Autodesk Fusion 360 part; units mm, degrees
(part 6 of 7)
  line L308 (64.4437, -54.0323) -> (64.499, -54.1149)
  line L309 (64.499, -54.1149) -> (64.5587, -54.1969)
  line L310 (64.5587, -54.1969) -> (64.6439, -54.1986)
  line L311 (64.6439, -54.1986) -> (64.7292, -54.1986)
  line L312 (64.7292, -54.1986) -> (64.8145, -54.1969)
  line L313 (64.8145, -54.1969) -> (64.8741, -54.1149)
  line L314 (64.8741, -54.1149) -> (64.9295, -54.0323)
  line L315 (64.9295, -54.0323) -> (64.9805, -53.949)
  line L316 (64.9805, -53.949) -> (65.027, -53.8654)
  line L317 (65.027, -53.8654) -> (65.069, -53.7814)
  line L318 (65.069, -53.7814) -> (65.1064, -53.6974)
  line L319 (65.1064, -53.6974) -> (65.1389, -53.6134)
  line L320 (65.1389, -53.6134) -> (65.1663, -53.5295)
  line L321 (65.1663, -53.5295) -> (65.1884, -53.4461)
  line L322 (65.1884, -53.4461) -> (65.2045, -53.3632)
  line L323 (65.2045, -53.3632) -> (65.2136, -53.2811)
  line L324 (65.2136, -53.2811) -> (65.2128, -53.2005)
  line L325 (65.2128, -53.2005) -> (65.1672, -52.9112)
  line L326 (65.1672, -52.9112) -> (65.3277, -52.8816)
  line L327 (65.3277, -52.8816) -> (65.4863, -52.8435)
  line L328 (65.4863, -52.8435) -> (65.6428, -52.7972)
  line L329 (65.6428, -52.7972) -> (65.7965, -52.7426)
  line L330 (65.7965, -52.7426) -> (65.9017, -53.0159)
  line L331 (65.9017, -53.0159) -> (65.9413, -53.0862)
  line L332 (65.9413, -53.0862) -> (65.9903, -53.1526)
  line L333 (65.9903, -53.1526) -> (66.0456, -53.2164)
  line L334 (66.0456, -53.2164) -> (66.1065, -53.2776)
  line L335 (66.1065, -53.2776) -> (66.1721, -53.3365)
  line L336 (66.1721, -53.3365) -> (66.2423, -53.393)
  line L337 (66.2423, -53.393) -> (66.3167, -53.4471)
  line L338 (66.3167, -53.4471) -> (66.395, -53.4988)
  line L339 (66.395, -53.4988) -> (66.4772, -53.548)
  line L340 (66.4772, -53.548) -> (66.563, -53.5946)
  line L341 (66.563, -53.5946) -> (66.6522, -53.6385)
  line L342 (66.6522, -53.6385) -> (66.7449, -53.6797)
  line L343 (66.7449, -53.6797) -> (66.8195, -53.6385)
  line L344 (66.8195, -53.6385) -> (66.8934, -53.5959)
  line L345 (66.8934, -53.5959) -> (66.9664, -53.5518)
  line L346 (66.9664, -53.5518) -> (66.9771, -53.451)
  line L347 (66.9771, -53.451) -> (66.9836, -53.3517)
  line L348 (66.9836, -53.3517) -> (66.9862, -53.2541)
  line L349 (66.9862, -53.2541) -> (66.9847, -53.1584)
  line L350 (66.9847, -53.1584) -> (66.9791, -53.0647)
  line L351 (66.9791, -53.0647) -> (66.9694, -52.9732)
  line L352 (66.9694, -52.9732) -> (66.9556, -52.8842)
  line L353 (66.9556, -52.8842) -> (66.9374, -52.7979)
  line L354 (66.9374, -52.7979) -> (66.9148, -52.7146)
  line L355 (66.9148, -52.7146) -> (66.8873, -52.6347)
  line L356 (66.8873, -52.6347) -> (66.8542, -52.5591)
  line L357 (66.8542, -52.5591) -> (66.8131, -52.4897)
  line L358 (66.8131, -52.4897) -> (66.629, -52.262)
  line L359 (66.629, -52.262) -> (66.7532, -52.1561)
  line L360 (66.7532, -52.1561) -> (66.8715, -52.0438)
  line L361 (66.8715, -52.0438) -> (66.9838, -51.9254)
  line L362 (66.9838, -51.9254) -> (67.0897, -51.8013)
  line L363 (67.0897, -51.8013) -> (67.3175, -51.9854)
  line L364 (67.3175, -51.9854) -> (67.3869, -52.0264)
  line L365 (67.3869, -52.0264) -> (67.4625, -52.0595)
  line L366 (67.4625, -52.0595) -> (67.5423, -52.087)
  line L367 (67.5423, -52.087) -> (67.6256, -52.1097)
  line L368 (67.6256, -52.1097) -> (67.712, -52.1278)
  line L369 (67.712, -52.1278) -> (67.801, -52.1417)
  line L370 (67.801, -52.1417) -> (67.8924, -52.1513)
  line L371 (67.8924, -52.1513) -> (67.9861, -52.1569)
  line L372 (67.9861, -52.1569) -> (68.0819, -52.1584)
  line L373 (68.0819, -52.1584) -> (68.1794, -52.1559)
  line L374 (68.1794, -52.1559) -> (68.2787, -52.1493)
  line L375 (68.2787, -52.1493) -> (68.3795, -52.1387)
  line L376 (68.3795, -52.1387) -> (68.4236, -52.0657)
  line L377 (68.4236, -52.0657) -> (68.4663, -51.9918)
  line L378 (68.4663, -51.9918) -> (68.5075, -51.9171)
  line L379 (68.5075, -51.9171) -> (68.4663, -51.8245)
  line L380 (68.4663, -51.8245) -> (68.4223, -51.7352)
  line L381 (68.4223, -51.7352) -> (68.3757, -51.6494)
  line L382 (68.3757, -51.6494) -> (68.3266, -51.5673)
  line L383 (68.3266, -51.5673) -> (68.2749, -51.4889)
  line L384 (68.2749, -51.4889) -> (68.2208, -51.4146)
  line L385 (68.2208, -51.4146) -> (68.1643, -51.3444)
  line L386 (68.1643, -51.3444) -> (68.1054, -51.2787)
  line L387 (68.1054, -51.2787) -> (68.0441, -51.2179)
  line L388 (68.0441, -51.2179) -> (67.9804, -51.1625)
  line L389 (67.9804, -51.1625) -> (67.9139, -51.1135)
  line L390 (67.9139, -51.1135) -> (67.8437, -51.074)
  line L391 (67.8437, -51.074) -> (67.5704, -50.9688)
  line L392 (67.5704, -50.9688) -> (67.6249, -50.815)
  line L393 (67.6249, -50.815) -> (67.6713, -50.6586)
  line L394 (67.6713, -50.6586) -> (67.7094, -50.4999)
  line L395 (67.7094, -50.4999) -> (67.739, -50.3395)
  circle A0 centre (64.6866, -49.8588) radius 1.5
extrude "Extrude2''" add sketch "Sketch2 (3)" along normal blind 2 separate body makes body 9 in component "CT idler 3"
combine "Combine1''" operation add target body 8 tool bodies 9 makes body 10 at (63.4191, -47.6635, 43.4) in component "CT idler 3"
ref_plane "WorkPlane1" through (0, 0, 43.4) normal (0, 0, 1) x (1, 0, 0) in component "CT dial wheel (tool body)"
sketch "Sketch1 (5)" plane through (0, 0, 43.4) normal (0, 0, 1) x (1, 0, 0) in component "CT dial wheel (tool body)"
  line L0 (77.4997, -64.3893) -> (77.838, -64.4048)
  line L1 (77.838, -64.4048) -> (77.9192, -64.4017)
  line L2 (77.9192, -64.4017) -> (78.0006, -64.3928)
  line L3 (78.0006, -64.3928) -> (78.0822, -64.3801)
  line L4 (78.0822, -64.3801) -> (78.1639, -64.3643)
  line L5 (78.1639, -64.3643) -> (78.2456, -64.3456)
  line L6 (78.2456, -64.3456) -> (78.3274, -64.3244)
  line L7 (78.3274, -64.3244) -> (78.4092, -64.3009)
  line L8 (78.4092, -64.3009) -> (78.491, -64.2751)
  line L9 (78.491, -64.2751) -> (78.5728, -64.2472)
  line L10 (78.5728, -64.2472) -> (78.6546, -64.2173)
  line L11 (78.6546, -64.2173) -> (78.7363, -64.1854)
  line L12 (78.7363, -64.1854) -> (78.818, -64.1516)
  line L13 (78.818, -64.1516) -> (78.8198, -64.0105)
  line L14 (78.8198, -64.0105) -> (78.8198, -63.8695)
  line L15 (78.8198, -63.8695) -> (78.818, -63.7284)
  line L16 (78.818, -63.7284) -> (78.7363, -63.6946)
  line L17 (78.7363, -63.6946) -> (78.6546, -63.6627)
  line L18 (78.6546, -63.6627) -> (78.5728, -63.6328)
  line L19 (78.5728, -63.6328) -> (78.491, -63.6049)
  line L20 (78.491, -63.6049) -> (78.4092, -63.5791)
  line L21 (78.4092, -63.5791) -> (78.3274, -63.5556)
  line L22 (78.3274, -63.5556) -> (78.2456, -63.5344)
  line L23 (78.2456, -63.5344) -> (78.1639, -63.5157)
  line L24 (78.1639, -63.5157) -> (78.0822, -63.4999)
  line L25 (78.0822, -63.4999) -> (78.0006, -63.4872)
  line L26 (78.0006, -63.4872) -> (77.9192, -63.4783)
  line L27 (77.9192, -63.4783) -> (77.838, -63.4752)
  line L28 (77.838, -63.4752) -> (77.4997, -63.4907)
  line L29 (77.4997, -63.4907) -> (77.4883, -63.2877)
  line L30 (77.4883, -63.2877) -> (77.4727, -63.085)
  line L31 (77.4727, -63.085) -> (77.4529, -62.8827)
  line L32 (77.4529, -62.8827) -> (77.4289, -62.6808)
  line L33 (77.4289, -62.6808) -> (77.7647, -62.6373)
  line L34 (77.7647, -62.6373) -> (77.8441, -62.6202)
  line L35 (77.8441, -62.6202) -> (77.9228, -62.5973)
  line L36 (77.9228, -62.5973) -> (78.0009, -62.5706)
  line L37 (78.0009, -62.5706) -> (78.0786, -62.5408)
  line L38 (78.0786, -62.5408) -> (78.1558, -62.5082)
  line L39 (78.1558, -62.5082) -> (78.2327, -62.4731)
  line L40 (78.2327, -62.4731) -> (78.3092, -62.4357)
  line L41 (78.3092, -62.4357) -> (78.3853, -62.3962)
  line L42 (78.3853, -62.3962) -> (78.461, -62.3545)
  line L43 (78.461, -62.3545) -> (78.5363, -62.3108)
  line L44 (78.5363, -62.3108) -> (78.6113, -62.2652)
  line L45 (78.6113, -62.2652) -> (78.6858, -62.2178)
  line L46 (78.6858, -62.2178) -> (78.6631, -62.0785)
  line L47 (78.6631, -62.0785) -> (78.6386, -61.9396)
  line L48 (78.6386, -61.9396) -> (78.6123, -61.801)
  line L49 (78.6123, -61.801) -> (78.526, -61.7819)
  line L50 (78.526, -61.7819) -> (78.44, -61.7647)
  line L51 (78.44, -61.7647) -> (78.3543, -61.7494)
  line L52 (78.3543, -61.7494) -> (78.2689, -61.7362)
  line L53 (78.2689, -61.7362) -> (78.1838, -61.725)
  line L54 (78.1838, -61.725) -> (78.0992, -61.716)
  line L55 (78.0992, -61.716) -> (78.015, -61.7093)
  line L56 (78.015, -61.7093) -> (77.9312, -61.7052)
  line L57 (77.9312, -61.7052) -> (77.848, -61.7037)
  line L58 (77.848, -61.7037) -> (77.7655, -61.7054)
  line L59 (77.7655, -61.7054) -> (77.6838, -61.7108)
  line L60 (77.6838, -61.7108) -> (77.6033, -61.7218)
  line L61 (77.6033, -61.7218) -> (77.2728, -61.7958)
  line L62 (77.2728, -61.7958) -> (77.2263, -61.5979)
  line L63 (77.2263, -61.5979) -> (77.1757, -61.401)
  line L64 (77.1757, -61.401) -> (77.1211, -61.2052)
  line L65 (77.1211, -61.2052) -> (77.0624, -61.0105)
  line L66 (77.0624, -61.0105) -> (77.3856, -60.9094)
  line L67 (77.3856, -60.9094) -> (77.4608, -60.8787)
  line L68 (77.4608, -60.8787) -> (77.5343, -60.8425)
  line L69 (77.5343, -60.8425) -> (77.6066, -60.8027)
  line L70 (77.6066, -60.8027) -> (77.6779, -60.7598)
  line L71 (77.6779, -60.7598) -> (77.7483, -60.7143)
  line L72 (77.7483, -60.7143) -> (77.818, -60.6664)
  line L73 (77.818, -60.6664) -> (77.8868, -60.6163)
  line L74 (77.8868, -60.6163) -> (77.9549, -60.5641)
  line L75 (77.9549, -60.5641) -> (78.0222, -60.5099)
  line L76 (78.0222, -60.5099) -> (78.0888, -60.4539)
  line L77 (78.0888, -60.4539) -> (78.1547, -60.396)
  line L78 (78.1547, -60.396) -> (78.2199, -60.3363)
  line L79 (78.2199, -60.3363) -> (78.1733, -60.2031)
  line L80 (78.1733, -60.2031) -> (78.125, -60.0705)
  line L81 (78.125, -60.0705) -> (78.0751, -59.9386)
  line L82 (78.0751, -59.9386) -> (77.9868, -59.9347)
  line L83 (77.9868, -59.9347) -> (77.8991, -59.9327)
  line L84 (77.8991, -59.9327) -> (77.8121, -59.9326)
  line L85 (77.8121, -59.9326) -> (77.7256, -59.9344)
  line L86 (77.7256, -59.9344) -> (77.6399, -59.9381)
  line L87 (77.6399, -59.9381) -> (77.555, -59.944)
  line L88 (77.555, -59.944) -> (77.4709, -59.9521)
  line L89 (77.4709, -59.9521) -> (77.3877, -59.9625)
  line L90 (77.3877, -59.9625) -> (77.3055, -59.9755)
  line L91 (77.3055, -59.9755) -> (77.2245, -59.9915)
  line L92 (77.2245, -59.9915) -> (77.145, -60.011)
  line L93 (77.145, -60.011) -> (77.0676, -60.0358)
  line L94 (77.0676, -60.0358) -> (76.755, -60.1661)
  line L95 (76.755, -60.1661) -> (76.6749, -59.9792)
  line L96 (76.6749, -59.9792) -> (76.5909, -59.7941)
  line L97 (76.5909, -59.7941) -> (76.5031, -59.6108)
  line L98 (76.5031, -59.6108) -> (76.4115, -59.4293)
  line L99 (76.4115, -59.4293) -> (76.7122, -59.2736)
  line L100 (76.7122, -59.2736) -> (76.7809, -59.2303)
  line L101 (76.7809, -59.2303) -> (76.847, -59.1819)
  line L102 (76.847, -59.1819) -> (76.9113, -59.1301)
  line L103 (76.9113, -59.1301) -> (76.9741, -59.0755)
  line L104 (76.9741, -59.0755) -> (77.0356, -59.0185)
  line L105 (77.0356, -59.0185) -> (77.0958, -58.9592)
  line L106 (77.0958, -58.9592) -> (77.1549, -58.8979)
  line L107 (77.1549, -58.8979) -> (77.2128, -58.8347)
  line L108 (77.2128, -58.8347) -> (77.2697, -58.7696)
  line L109 (77.2697, -58.7696) -> (77.3256, -58.7028)
  line L110 (77.3256, -58.7028) -> (77.3804, -58.6344)
  line L111 (77.3804, -58.6344) -> (77.4343, -58.5643)
  line L112 (77.4343, -58.5643) -> (77.3653, -58.4412)
  line L113 (77.3653, -58.4412) -> (77.2947, -58.319)
  line L114 (77.2947, -58.319) -> (77.2226, -58.1977)
  line L115 (77.2226, -58.1977) -> (77.135, -58.2093)
  line L116 (77.135, -58.2093) -> (77.0483, -58.2226)
  line L117 (77.0483, -58.2226) -> (76.9625, -58.2375)
  line L118 (76.9625, -58.2375) -> (76.8778, -58.2543)
  line L119 (76.8778, -58.2543) -> (76.794, -58.2729)
  line L120 (76.794, -58.2729) -> (76.7114, -58.2934)
  line L121 (76.7114, -58.2934) -> (76.63, -58.3159)
  line L122 (76.63, -58.3159) -> (76.5498, -58.3407)
  line L123 (76.5498, -58.3407) -> (76.4712, -58.3677)
  line L124 (76.4712, -58.3677) -> (76.3942, -58.3975)
  line L125 (76.3942, -58.3975) -> (76.3192, -58.4305)
  line L126 (76.3192, -58.4305) -> (76.2474, -58.4684)
  line L127 (76.2474, -58.4684) -> (75.9621, -58.651)
  line L128 (75.9621, -58.651) -> (75.8508, -58.4809)
  line L129 (75.8508, -58.4809) -> (75.7359, -58.3132)
  line L130 (75.7359, -58.3132) -> (75.6176, -58.1479)
  line L131 (75.6176, -58.1479) -> (75.4958, -57.9851)
  line L132 (75.4958, -57.9851) -> (75.765, -57.7795)
  line L133 (75.765, -57.7795) -> (75.8251, -57.7249)
  line L134 (75.8251, -57.7249) -> (75.8818, -57.6658)
  line L135 (75.8818, -57.6658) -> (75.9361, -57.6036)
  line L136 (75.9361, -57.6036) -> (75.9885, -57.539)
  line L137 (75.9885, -57.539) -> (76.0391, -57.4721)
  line L138 (76.0391, -57.4721) -> (76.0881, -57.4033)
  line L139 (76.0881, -57.4033) -> (76.1357, -57.3327)
  line L140 (76.1357, -57.3327) -> (76.1818, -57.2604)
  line L141 (76.1818, -57.2604) -> (76.2265, -57.1864)
  line L142 (76.2265, -57.1864) -> (76.2699, -57.1109)
  line L143 (76.2699, -57.1109) -> (76.3121, -57.034)
  line L144 (76.3121, -57.034) -> (76.3529, -56.9556)
  line L145 (76.3529, -56.9556) -> (76.2636, -56.8464)
  line L146 (76.2636, -56.8464) -> (76.1729, -56.7383)
  line L147 (76.1729, -56.7383) -> (76.0808, -56.6314)
  line L148 (76.0808, -56.6314) -> (75.9966, -56.658)
  line L149 (75.9966, -56.658) -> (75.9135, -56.6861)
  line L150 (75.9135, -56.6861) -> (75.8316, -56.7158)
  line L151 (75.8316, -56.7158) -> (75.751, -56.747)
  line L152 (75.751, -56.747) -> (75.6718, -56.7798)
  line L153 (75.6718, -56.7798) -> (75.594, -56.8144)
  line L154 (75.594, -56.8144) -> (75.5177, -56.8507)
  line L155 (75.5177, -56.8507) -> (75.4431, -56.889)
  line L156 (75.4431, -56.889) -> (75.3703, -56.9293)
  line L157 (75.3703, -56.9293) -> (75.2997, -56.972)
  line L158 (75.2997, -56.972) -> (75.2316, -57.0175)
  line L159 (75.2316, -57.0175) -> (75.1674, -57.0673)
  line L160 (75.1674, -57.0673) -> (74.9182, -57.2967)
  line L161 (74.9182, -57.2967) -> (74.779, -57.1485)
  line L162 (74.779, -57.1485) -> (74.6367, -57.0033)
  line L163 (74.6367, -57.0033) -> (74.4915, -56.861)
  line L164 (74.4915, -56.861) -> (74.3433, -56.7218)
  line L165 (74.3433, -56.7218) -> (74.5727, -56.4726)
  line L166 (74.5727, -56.4726) -> (74.6225, -56.4084)
  line L167 (74.6225, -56.4084) -> (74.668, -56.3403)
  line L168 (74.668, -56.3403) -> (74.7107, -56.2697)
  line L169 (74.7107, -56.2697) -> (74.751, -56.1969)
  line L170 (74.751, -56.1969) -> (74.7893, -56.1223)
  line L171 (74.7893, -56.1223) -> (74.8256, -56.046)
  line L172 (74.8256, -56.046) -> (74.8602, -55.9682)
  line L173 (74.8602, -55.9682) -> (74.893, -55.889)
  line L174 (74.893, -55.889) -> (74.9242, -55.8084)
  line L175 (74.9242, -55.8084) -> (74.9539, -55.7265)
  line L176 (74.9539, -55.7265) -> (74.982, -55.6434)
  line L177 (74.982, -55.6434) -> (75.0086, -55.5592)
  line L178 (75.0086, -55.5592) -> (74.9017, -55.4671)
  line L179 (74.9017, -55.4671) -> (74.7936, -55.3764)
  line L180 (74.7936, -55.3764) -> (74.6844, -55.2871)
  line L181 (74.6844, -55.2871) -> (74.606, -55.3279)
  line L182 (74.606, -55.3279) -> (74.5291, -55.3701)
  line L183 (74.5291, -55.3701) -> (74.4536, -55.4135)
  line L184 (74.4536, -55.4135) -> (74.3796, -55.4582)
  line L185 (74.3796, -55.4582) -> (74.3073, -55.5043)
  line L186 (74.3073, -55.5043) -> (74.2367, -55.5519)
  line L187 (74.2367, -55.5519) -> (74.1679, -55.6009)
  line L188 (74.1679, -55.6009) -> (74.101, -55.6515)
  line L189 (74.101, -55.6515) -> (74.0364, -55.7039)
  line L190 (74.0364, -55.7039) -> (73.9742, -55.7582)
  line L191 (73.9742, -55.7582) -> (73.9151, -55.8149)
  line L192 (73.9151, -55.8149) -> (73.8605, -55.875)
  line L193 (73.8605, -55.875) -> (73.6549, -56.1442)
  line L194 (73.6549, -56.1442) -> (73.4921, -56.0224)
  line L195 (73.4921, -56.0224) -> (73.3268, -55.9041)
  line L196 (73.3268, -55.9041) -> (73.1591, -55.7892)
  line L197 (73.1591, -55.7892) -> (72.989, -55.6779)
  line L198 (72.989, -55.6779) -> (73.1716, -55.3926)
  line L199 (73.1716, -55.3926) -> (73.2095, -55.3208)
  line L200 (73.2095, -55.3208) -> (73.2425, -55.2458)
  line L201 (73.2425, -55.2458) -> (73.2723, -55.1688)
  line L202 (73.2723, -55.1688) -> (73.2993, -55.0902)
  line L203 (73.2993, -55.0902) -> (73.3241, -55.01)
  line L204 (73.3241, -55.01) -> (73.3466, -54.9286)
  line L205 (73.3466, -54.9286) -> (73.3671, -54.846)
  line L206 (73.3671, -54.846) -> (73.3857, -54.7622)
  line L207 (73.3857, -54.7622) -> (73.4025, -54.6775)
  line L208 (73.4025, -54.6775) -> (73.4174, -54.5917)
  line L209 (73.4174, -54.5917) -> (73.4307, -54.505)
  line L210 (73.4307, -54.505) -> (73.4423, -54.4174)
  line L211 (73.4423, -54.4174) -> (73.321, -54.3453)
  line L212 (73.321, -54.3453) -> (73.1988, -54.2747)
  line L213 (73.1988, -54.2747) -> (73.0757, -54.2057)
  line L214 (73.0757, -54.2057) -> (73.0056, -54.2596)
  line L215 (73.0056, -54.2596) -> (72.9372, -54.3144)
  line L216 (72.9372, -54.3144) -> (72.8704, -54.3703)
  line L217 (72.8704, -54.3703) -> (72.8053, -54.4272)
  line L218 (72.8053, -54.4272) -> (72.7421, -54.4851)
  line L219 (72.7421, -54.4851) -> (72.6808, -54.5442)
  line L220 (72.6808, -54.5442) -> (72.6215, -54.6044)
  line L221 (72.6215, -54.6044) -> (72.5645, -54.6659)
  line L222 (72.5645, -54.6659) -> (72.5099, -54.7287)
  line L223 (72.5099, -54.7287) -> (72.4581, -54.793)
  line L224 (72.4581, -54.793) -> (72.4097, -54.8591)
  line L225 (72.4097, -54.8591) -> (72.3664, -54.9278)
  line L226 (72.3664, -54.9278) -> (72.2107, -55.2285)
  line L227 (72.2107, -55.2285) -> (72.0292, -55.1369)
  line L228 (72.0292, -55.1369) -> (71.8459, -55.0491)
  line L229 (71.8459, -55.0491) -> (71.6608, -54.9651)
  line L230 (71.6608, -54.9651) -> (71.4739, -54.885)
  line L231 (71.4739, -54.885) -> (71.6042, -54.5724)
  line L232 (71.6042, -54.5724) -> (71.629, -54.495)
  line L233 (71.629, -54.495) -> (71.6485, -54.4155)
  line L234 (71.6485, -54.4155) -> (71.6645, -54.3345)
  line L235 (71.6645, -54.3345) -> (71.6775, -54.2523)
  line L236 (71.6775, -54.2523) -> (71.6879, -54.1691)
  line L237 (71.6879, -54.1691) -> (71.696, -54.085)
  line L238 (71.696, -54.085) -> (71.7019, -54.0001)
  line L239 (71.7019, -54.0001) -> (71.7056, -53.9144)
  line L240 (71.7056, -53.9144) -> (71.7074, -53.8279)
  line L241 (71.7074, -53.8279) -> (71.7073, -53.7409)
  line L242 (71.7073, -53.7409) -> (71.7053, -53.6532)
  line L243 (71.7053, -53.6532) -> (71.7014, -53.5649)
  line L244 (71.7014, -53.5649) -> (71.5695, -53.515)
  line L245 (71.5695, -53.515) -> (71.4369, -53.4667)
  line L246 (71.4369, -53.4667) -> (71.3037, -53.4201)
  line L247 (71.3037, -53.4201) -> (71.244, -53.4853)
  line L248 (71.244, -53.4853) -> (71.1861, -53.5512)
  line L249 (71.1861, -53.5512) -> (71.1301, -53.6178)
  line L250 (71.1301, -53.6178) -> (71.0759, -53.6851)
  line L251 (71.0759, -53.6851) -> (71.0237, -53.7532)
  line L252 (71.0237, -53.7532) -> (70.9736, -53.822)
  line L253 (70.9736, -53.822) -> (70.9257, -53.8917)
  line L254 (70.9257, -53.8917) -> (70.8802, -53.9621)
  line L255 (70.8802, -53.9621) -> (70.8373, -54.0334)
  line L256 (70.8373, -54.0334) -> (70.7975, -54.1057)
  line L257 (70.7975, -54.1057) -> (70.7613, -54.1792)
  line L258 (70.7613, -54.1792) -> (70.7306, -54.2544)
  line L259 (70.7306, -54.2544) -> (70.6295, -54.5776)
  line L260 (70.6295, -54.5776) -> (70.4348, -54.5189)
  line L261 (70.4348, -54.5189) -> (70.239, -54.4643)
  line L262 (70.239, -54.4643) -> (70.0421, -54.4137)
  line L263 (70.0421, -54.4137) -> (69.8442, -54.3672)
  line L264 (69.8442, -54.3672) -> (69.9182, -54.0367)
  line L265 (69.9182, -54.0367) -> (69.9292, -53.9562)
  line L266 (69.9292, -53.9562) -> (69.9346, -53.8745)
  line L267 (69.9346, -53.8745) -> (69.9363, -53.792)
  line L268 (69.9363, -53.792) -> (69.9348, -53.7088)
  line L269 (69.9348, -53.7088) -> (69.9307, -53.625)
  line L270 (69.9307, -53.625) -> (69.924, -53.5408)
  line L271 (69.924, -53.5408) -> (69.915, -53.4562)
  line L272 (69.915, -53.4562) -> (69.9038, -53.3711)
  line L273 (69.9038, -53.3711) -> (69.8906, -53.2857)
  line L274 (69.8906, -53.2857) -> (69.8753, -53.2)
  line L275 (69.8753, -53.2) -> (69.8581, -53.114)
  line L276 (69.8581, -53.114) -> (69.839, -53.0277)
  line L277 (69.839, -53.0277) -> (69.7004, -53.0014)
  line L278 (69.7004, -53.0014) -> (69.5615, -52.9769)
  line L279 (69.5615, -52.9769) -> (69.4222, -52.9542)
  line L280 (69.4222, -52.9542) -> (69.3748, -53.0287)
  line L281 (69.3748, -53.0287) -> (69.3292, -53.1037)
  line L282 (69.3292, -53.1037) -> (69.2855, -53.179)
  line L283 (69.2855, -53.179) -> (69.2438, -53.2547)
  line L284 (69.2438, -53.2547) -> (69.2043, -53.3308)
  line L285 (69.2043, -53.3308) -> (69.1669, -53.4073)
  line L286 (69.1669, -53.4073) -> (69.1318, -53.4842)
  line L287 (69.1318, -53.4842) -> (69.0992, -53.5614)
  line L288 (69.0992, -53.5614) -> (69.0694, -53.6391)
  line L289 (69.0694, -53.6391) -> (69.0427, -53.7172)
  line L290 (69.0427, -53.7172) -> (69.0198, -53.7959)
  line L291 (69.0198, -53.7959) -> (69.0027, -53.8753)
  line L292 (69.0027, -53.8753) -> (68.9592, -54.2111)
  line L293 (68.9592, -54.2111) -> (68.7573, -54.1871)
  line L294 (68.7573, -54.1871) -> (68.555, -54.1673)
  line L295 (68.555, -54.1673) -> (68.3523, -54.1517)
  line L296 (68.3523, -54.1517) -> (68.1493, -54.1403)
  line L297 (68.1493, -54.1403) -> (68.1648, -53.802)
  line L298 (68.1648, -53.802) -> (68.1617, -53.7208)
  line L299 (68.1617, -53.7208) -> (68.1528, -53.6394)
  line L300 (68.1528, -53.6394) -> (68.1401, -53.5578)
  line L301 (68.1401, -53.5578) -> (68.1243, -53.4761)
  line L302 (68.1243, -53.4761) -> (68.1056, -53.3944)
  line L303 (68.1056, -53.3944) -> (68.0844, -53.3126)
  line L304 (68.0844, -53.3126) -> (68.0609, -53.2308)
  line L305 (68.0609, -53.2308) -> (68.0351, -53.149)
  line L306 (68.0351, -53.149) -> (68.0072, -53.0672)
  line L307 (68.0072, -53.0672) -> (67.9773, -52.9854)
  line L308 (67.9773, -52.9854) -> (67.9454, -52.9037)
  line L309 (67.9454, -52.9037) -> (67.9116, -52.822)
  line L310 (67.9116, -52.822) -> (67.7705, -52.8202)
  line L311 (67.7705, -52.8202) -> (67.6295, -52.8202)
  line L312 (67.6295, -52.8202) -> (67.4884, -52.822)
  line L313 (67.4884, -52.822) -> (67.4546, -52.9037)
  line L314 (67.4546, -52.9037) -> (67.4227, -52.9854)
  line L315 (67.4227, -52.9854) -> (67.3928, -53.0672)
  line L316 (67.3928, -53.0672) -> (67.3649, -53.149)
  line L317 (67.3649, -53.149) -> (67.3391, -53.2308)
  line L318 (67.3391, -53.2308) -> (67.3156, -53.3126)
  line L319 (67.3156, -53.3126) -> (67.2944, -53.3944)
  line L320 (67.2944, -53.3944) -> (67.2757, -53.4761)
  line L321 (67.2757, -53.4761) -> (67.2599, -53.5578)
  line L322 (67.2599, -53.5578) -> (67.2472, -53.6394)
  line L323 (67.2472, -53.6394) -> (67.2383, -53.7208)
  line L324 (67.2383, -53.7208) -> (67.2352, -53.802)
  line L325 (67.2352, -53.802) -> (67.2507, -54.1403)
  line L326 (67.2507, -54.1403) -> (67.0477, -54.1517)
  line L327 (67.0477, -54.1517) -> (66.845, -54.1673)
  line L328 (66.845, -54.1673) -> (66.6427, -54.1871)
  line L329 (66.6427, -54.1871) -> (66.4408, -54.2111)
  line L330 (66.4408, -54.2111) -> (66.3973, -53.8753)
  line L331 (66.3973, -53.8753) -> (66.3802, -53.7959)
  line L332 (66.3802, -53.7959) -> (66.3573, -53.7172)
  line L333 (66.3573, -53.7172) -> (66.3306, -53.6391)
  line L334 (66.3306, -53.6391) -> (66.3008, -53.5614)
  line L335 (66.3008, -53.5614) -> (66.2682, -53.4842)
  line L336 (66.2682, -53.4842) -> (66.2331, -53.4073)
  line L337 (66.2331, -53.4073) -> (66.1957, -53.3308)
  line L338 (66.1957, -53.3308) -> (66.1562, -53.2547)
  line L339 (66.1562, -53.2547) -> (66.1145, -53.179)
  line L340 (66.1145, -53.179) -> (66.0708, -53.1037)
  line L341 (66.0708, -53.1037) -> (66.0252, -53.0287)
  line L342 (66.0252, -53.0287) -> (65.9778, -52.9542)
  line L343 (65.9778, -52.9542) -> (65.8385, -52.9769)
  line L344 (65.8385, -52.9769) -> (65.6996, -53.0014)
  line L345 (65.6996, -53.0014) -> (65.561, -53.0277)
  line L346 (65.561, -53.0277) -> (65.5419, -53.114)
  line L347 (65.5419, -53.114) -> (65.5247, -53.2)
  line L348 (65.5247, -53.2) -> (65.5094, -53.2857)
  line L349 (65.5094, -53.2857) -> (65.4962, -53.3711)
  line L350 (65.4962, -53.3711) -> (65.485, -53.4562)
  line L351 (65.485, -53.4562) -> (65.476, -53.5408)
  line L352 (65.476, -53.5408) -> (65.4693, -53.625)
  line L353 (65.4693, -53.625) -> (65.4652, -53.7088)
  line L354 (65.4652, -53.7088) -> (65.4637, -53.792)
  line L355 (65.4637, -53.792) -> (65.4654, -53.8745)
  line L356 (65.4654, -53.8745) -> (65.4708, -53.9562)
  line L357 (65.4708, -53.9562) -> (65.4818, -54.0367)
  line L358 (65.4818, -54.0367) -> (65.5558, -54.3672)
  line L359 (65.5558, -54.3672) -> (65.3579, -54.4137)
  line L360 (65.3579, -54.4137) -> (65.161, -54.4643)
  line L361 (65.161, -54.4643) -> (64.9652, -54.5189)
  line L362 (64.9652, -54.5189) -> (64.7705, -54.5776)
  line L363 (64.7705, -54.5776) -> (64.6694, -54.2544)
  line L364 (64.6694, -54.2544) -> (64.6387, -54.1792)
  line L365 (64.6387, -54.1792) -> (64.6025, -54.1057)
  line L366 (64.6025, -54.1057) -> (64.5627, -54.0334)
  line L367 (64.5627, -54.0334) -> (64.5198, -53.9621)
  line L368 (64.5198, -53.9621) -> (64.4743, -53.8917)
  line L369 (64.4743, -53.8917) -> (64.4264, -53.822)
  line L370 (64.4264, -53.822) -> (64.3763, -53.7532)
  line L371 (64.3763, -53.7532) -> (64.3241, -53.6851)
  line L372 (64.3241, -53.6851) -> (64.2699, -53.6178)
  line L373 (64.2699, -53.6178) -> (64.2139, -53.5512)
  line L374 (64.2139, -53.5512) -> (64.156, -53.4853)
  line L375 (64.156, -53.4853) -> (64.0963, -53.4201)
  line L376 (64.0963, -53.4201) -> (63.9631, -53.4667)
  line L377 (63.9631, -53.4667) -> (63.8305, -53.515)
  line L378 (63.8305, -53.515) -> (63.6986, -53.5649)
  line L379 (63.6986, -53.5649) -> (63.6947, -53.6532)
  line L380 (63.6947, -53.6532) -> (63.6927, -53.7409)
  line L381 (63.6927, -53.7409) -> (63.6926, -53.8279)
  line L382 (63.6926, -53.8279) -> (63.6944, -53.9144)
  line L383 (63.6944, -53.9144) -> (63.6981, -54.0001)
  line L384 (63.6981, -54.0001) -> (63.704, -54.085)
  line L385 (63.704, -54.085) -> (63.7121, -54.1691)
  line L386 (63.7121, -54.1691) -> (63.7225, -54.2523)
  line L387 (63.7225, -54.2523) -> (63.7355, -54.3345)
  line L388 (63.7355, -54.3345) -> (63.7515, -54.4155)
  line L389 (63.7515, -54.4155) -> (63.771, -54.495)
  line L390 (63.771, -54.495) -> (63.7958, -54.5724)
  line L391 (63.7958, -54.5724) -> (63.9261, -54.885)
  line L392 (63.9261, -54.885) -> (63.7392, -54.9651)
  line L393 (63.7392, -54.9651) -> (63.5541, -55.0491)
  line L394 (63.5541, -55.0491) -> (63.3708, -55.1369)
  line L395 (63.3708, -55.1369) -> (63.1893, -55.2285)
  line L396 (63.1893, -55.2285) -> (63.0336, -54.9278)
  line L397 (63.0336, -54.9278) -> (62.9903, -54.8591)
  line L398 (62.9903, -54.8591) -> (62.9419, -54.793)
  line L399 (62.9419, -54.793) -> (62.8901, -54.7287)
  line L400 (62.8901, -54.7287) -> (62.8355, -54.6659)
  line L401 (62.8355, -54.6659) -> (62.7785, -54.6044)
  line L402 (62.7785, -54.6044) -> (62.7192, -54.5442)
  line L403 (62.7192, -54.5442) -> (62.6579, -54.4851)
  line L404 (62.6579, -54.4851) -> (62.5947, -54.4272)
  line L405 (62.5947, -54.4272) -> (62.5296, -54.3703)
  line L406 (62.5296, -54.3703) -> (62.4628, -54.3144)
  line L407 (62.4628, -54.3144) -> (62.3944, -54.2596)
  line L408 (62.3944, -54.2596) -> (62.3243, -54.2057)
  line L409 (62.3243, -54.2057) -> (62.2012, -54.2747)
  line L410 (62.2012, -54.2747) -> (62.079, -54.3453)
  line L411 (62.079, -54.3453) -> (61.9577, -54.4174)
  line L412 (61.9577, -54.4174) -> (61.9693, -54.505)
  line L413 (61.9693, -54.505) -> (61.9826, -54.5917)
  line L414 (61.9826, -54.5917) -> (61.9975, -54.6775)
  line L415 (61.9975, -54.6775) -> (62.0143, -54.7622)
  line L416 (62.0143, -54.7622) -> (62.0329, -54.846)
  line L417 (62.0329, -54.846) -> (62.0534, -54.9286)
  line L418 (62.0534, -54.9286) -> (62.0759, -55.01)
  line L419 (62.0759, -55.01) -> (62.1007, -55.0902)
  line L420 (62.1007, -55.0902) -> (62.1277, -55.1688)
  line L421 (62.1277, -55.1688) -> (62.1575, -55.2458)
  line L422 (62.1575, -55.2458) -> (62.1905, -55.3208)
  line L423 (62.1905, -55.3208) -> (62.2284, -55.3926)
  line L424 (62.2284, -55.3926) -> (62.411, -55.6779)
  line L425 (62.411, -55.6779) -> (62.2409, -55.7892)
  line L426 (62.2409, -55.7892) -> (62.0732, -55.9041)
  line L427 (62.0732, -55.9041) -> (61.9079, -56.0224)
  line L428 (61.9079, -56.0224) -> (61.7451, -56.1442)
  line L429 (61.7451, -56.1442) -> (61.5395, -55.875)
  line L430 (61.5395, -55.875) -> (61.4849, -55.8149)
  line L431 (61.4849, -55.8149) -> (61.4258, -55.7582)
  line L432 (61.4258, -55.7582) -> (61.3636, -55.7039)
  line L433 (61.3636, -55.7039) -> (61.299, -55.6515)
  line L434 (61.299, -55.6515) -> (61.2321, -55.6009)
  line L435 (61.2321, -55.6009) -> (61.1633, -55.5519)
  line L436 (61.1633, -55.5519) -> (61.0927, -55.5043)
  line L437 (61.0927, -55.5043) -> (61.0204, -55.4582)
  line L438 (61.0204, -55.4582) -> (60.9464, -55.4135)
  line L439 (60.9464, -55.4135) -> (60.8709, -55.3701)
  line L440 (60.8709, -55.3701) -> (60.794, -55.3279)
  line L441 (60.794, -55.3279) -> (60.7156, -55.2871)
  line L442 (60.7156, -55.2871) -> (60.6064, -55.3764)
  line L443 (60.6064, -55.3764) -> (60.4983, -55.4671)
  line L444 (60.4983, -55.4671) -> (60.3914, -55.5592)
  line L445 (60.3914, -55.5592) -> (60.418, -55.6434)
  line L446 (60.418, -55.6434) -> (60.4461, -55.7265)
  line L447 (60.4461, -55.7265) -> (60.4758, -55.8084)
  line L448 (60.4758, -55.8084) -> (60.507, -55.889)
  line L449 (60.507, -55.889) -> (60.5398, -55.9682)
  line L450 (60.5398, -55.9682) -> (60.5744, -56.046)
  line L451 (60.5744, -56.046) -> (60.6107, -56.1223)
  line L452 (60.6107, -56.1223) -> (60.649, -56.1969)
  line L453 (60.649, -56.1969) -> (60.6893, -56.2697)
  line L454 (60.6893, -56.2697) -> (60.732, -56.3403)
  line L455 (60.732, -56.3403) -> (60.7775, -56.4084)
  line L456 (60.7775, -56.4084) -> (60.8273, -56.4726)
  line L457 (60.8273, -56.4726) -> (61.0567, -56.7218)
  line L458 (61.0567, -56.7218) -> (60.9085, -56.861)
  line L459 (60.9085, -56.861) -> (60.7633, -57.0033)
  line L460 (60.7633, -57.0033) -> (60.621, -57.1485)
  line L461 (60.621, -57.1485) -> (60.4818, -57.2967)
  line L462 (60.4818, -57.2967) -> (60.2326, -57.0673)
  line L463 (60.2326, -57.0673) -> (60.1684, -57.0175)
  line L464 (60.1684, -57.0175) -> (60.1003, -56.972)
  line L465 (60.1003, -56.972) -> (60.0297, -56.9293)
  line L466 (60.0297, -56.9293) -> (59.9569, -56.889)
  line L467 (59.9569, -56.889) -> (59.8823, -56.8507)
  line L468 (59.8823, -56.8507) -> (59.806, -56.8144)
  line L469 (59.806, -56.8144) -> (59.7282, -56.7798)
  line L470 (59.7282, -56.7798) -> (59.649, -56.747)
  line L471 (59.649, -56.747) -> (59.5684, -56.7158)
  line L472 (59.5684, -56.7158) -> (59.4865, -56.6861)
  line L473 (59.4865, -56.6861) -> (59.4034, -56.658)
  line L474 (59.4034, -56.658) -> (59.3192, -56.6314)
  line L475 (59.3192, -56.6314) -> (59.2271, -56.7383)
  line L476 (59.2271, -56.7383) -> (59.1364, -56.8464)
  line L477 (59.1364, -56.8464) -> (59.0471, -56.9556)
  line L478 (59.0471, -56.9556) -> (59.0879, -57.034)
  line L479 (59.0879, -57.034) -> (59.1301, -57.1109)
  line L480 (59.1301, -57.1109) -> (59.1735, -57.1864)
  line L481 (59.1735, -57.1864) -> (59.2182, -57.2604)
  line L482 (59.2182, -57.2604) -> (59.2643, -57.3327)
  line L483 (59.2643, -57.3327) -> (59.3119, -57.4033)
  line L484 (59.3119, -57.4033) -> (59.3609, -57.4721)
  line L485 (59.3609, -57.4721) -> (59.4115, -57.539)
  line L486 (59.4115, -57.539) -> (59.4639, -57.6036)
  line L487 (59.4639, -57.6036) -> (59.5182, -57.6658)
  line L488 (59.5182, -57.6658) -> (59.5749, -57.7249)
  line L489 (59.5749, -57.7249) -> (59.635, -57.7795)
  line L490 (59.635, -57.7795) -> (59.9042, -57.9851)
  line L491 (59.9042, -57.9851) -> (59.7824, -58.1479)
  line L492 (59.7824, -58.1479) -> (59.6641, -58.3132)
  line L493 (59.6641, -58.3132) -> (59.5492, -58.4809)
  line L494 (59.5492, -58.4809) -> (59.4379, -58.651)
  line L495 (59.4379, -58.651) -> (59.1526, -58.4684)
  line L496 (59.1526, -58.4684) -> (59.0808, -58.4305)
  line L497 (59.0808, -58.4305) -> (59.0058, -58.3975)
  line L498 (59.0058, -58.3975) -> (58.9288, -58.3677)
  line L499 (58.9288, -58.3677) -> (58.8502, -58.3407)
  line L500 (58.8502, -58.3407) -> (58.77, -58.3159)
  line L501 (58.77, -58.3159) -> (58.6886, -58.2934)
  line L502 (58.6886, -58.2934) -> (58.606, -58.2729)
  line L503 (58.606, -58.2729) -> (58.5222, -58.2543)
  line L504 (58.5222, -58.2543) -> (58.4375, -58.2375)
  line L505 (58.4375, -58.2375) -> (58.3517, -58.2226)
  line L506 (58.3517, -58.2226) -> (58.265, -58.2093)
  line L507 (58.265, -58.2093) -> (58.1774, -58.1977)
  line L508 (58.1774, -58.1977) -> (58.1053, -58.319)
  line L509 (58.1053, -58.319) -> (58.0347, -58.4412)
  line L510 (58.0347, -58.4412) -> (57.9657, -58.5643)
  line L511 (57.9657, -58.5643) -> (58.0196, -58.6344)
  line L512 (58.0196, -58.6344) -> (58.0744, -58.7028)
  line L513 (58.0744, -58.7028) -> (58.1303, -58.7696)
  line L514 (58.1303, -58.7696) -> (58.1872, -58.8347)
  line L515 (58.1872, -58.8347) -> (58.2451, -58.8979)
  line L516 (58.2451, -58.8979) -> (58.3042, -58.9592)
  line L517 (58.3042, -58.9592) -> (58.3644, -59.0185)
  line L518 (58.3644, -59.0185) -> (58.4259, -59.0755)
  line L519 (58.4259, -59.0755) -> (58.4887, -59.1301)
  line L520 (58.4887, -59.1301) -> (58.553, -59.1819)
  line L521 (58.553, -59.1819) -> (58.6191, -59.2303)
  line L522 (58.6191, -59.2303) -> (58.6878, -59.2736)
  line L523 (58.6878, -59.2736) -> (58.9885, -59.4293)
  line L524 (58.9885, -59.4293) -> (58.8969, -59.6108)
  line L525 (58.8969, -59.6108) -> (58.8091, -59.7941)
  line L526 (58.8091, -59.7941) -> (58.7251, -59.9792)
  line L527 (58.7251, -59.9792) -> (58.645, -60.1661)
  line L528 (58.645, -60.1661) -> (58.3324, -60.0358)
  line L529 (58.3324, -60.0358) -> (58.255, -60.011)
  line L530 (58.255, -60.011) -> (58.1755, -59.9915)
  line L531 (58.1755, -59.9915) -> (58.0945, -59.9755)
  line L532 (58.0945, -59.9755) -> (58.0123, -59.9625)
  line L533 (58.0123, -59.9625) -> (57.9291, -59.9521)
  line L534 (57.9291, -59.9521) -> (57.845, -59.944)
  line L535 (57.845, -59.944) -> (57.7601, -59.9381)
  line L536 (57.7601, -59.9381) -> (57.6744, -59.9344)
  line L537 (57.6744, -59.9344) -> (57.5879, -59.9326)
  line L538 (57.5879, -59.9326) -> (57.5009, -59.9327)
  line L539 (57.5009, -59.9327) -> (57.4132, -59.9347)
  line L540 (57.4132, -59.9347) -> (57.3249, -59.9386)
  line L541 (57.3249, -59.9386) -> (57.275, -60.0705)
  line L542 (57.275, -60.0705) -> (57.2267, -60.2031)
  line L543 (57.2267, -60.2031) -> (57.1801, -60.3363)
  line L544 (57.1801, -60.3363) -> (57.2453, -60.396)
  line L545 (57.2453, -60.396) -> (57.3112, -60.4539)
  line L546 (57.3112, -60.4539) -> (57.3778, -60.5099)
  line L547 (57.3778, -60.5099) -> (57.4451, -60.5641)
  line L548 (57.4451, -60.5641) -> (57.5132, -60.6163)
  line L549 (57.5132, -60.6163) -> (57.582, -60.6664)
  line L550 (57.582, -60.6664) -> (57.6517, -60.7143)
  line L551 (57.6517, -60.7143) -> (57.7221, -60.7598)
  line L552 (57.7221, -60.7598) -> (57.7934, -60.8027)
  line L553 (57.7934, -60.8027) -> (57.8657, -60.8425)
  line L554 (57.8657, -60.8425) -> (57.9392, -60.8787)
  line L555 (57.9392, -60.8787) -> (58.0144, -60.9094)
  line L556 (58.0144, -60.9094) -> (58.3376, -61.0105)
  line L557 (58.3376, -61.0105) -> (58.2789, -61.2052)
  line L558 (58.2789, -61.2052) -> (58.2243, -61.401)
  line L559 (58.2243, -61.401) -> (58.1737, -61.5979)
  line L560 (58.1737, -61.5979) -> (58.1272, -61.7958)
  line L561 (58.1272, -61.7958) -> (57.7967, -61.7218)
  line L562 (57.7967, -61.7218) -> (57.7162, -61.7108)
  line L563 (57.7162, -61.7108) -> (57.6345, -61.7054)
  line L564 (57.6345, -61.7054) -> (57.552, -61.7037)
  line L565 (57.552, -61.7037) -> (57.4688, -61.7052)
  line L566 (57.4688, -61.7052) -> (57.385, -61.7093)
  line L567 (57.385, -61.7093) -> (57.3008, -61.716)
  line L568 (57.3008, -61.716) -> (57.2162, -61.725)
  line L569 (57.2162, -61.725) -> (57.1311, -61.7362)
  line L570 (57.1311, -61.7362) -> (57.0457, -61.7494)
  line L571 (57.0457, -61.7494) -> (56.96, -61.7647)
  line L572 (56.96, -61.7647) -> (56.874, -61.7819)
  line L573 (56.874, -61.7819) -> (56.7877, -61.801)
  line L574 (56.7877, -61.801) -> (56.7614, -61.9396)
  line L575 (56.7614, -61.9396) -> (56.7369, -62.0785)
  line L576 (56.7369, -62.0785) -> (56.7142, -62.2178)
  line L577 (56.7142, -62.2178) -> (56.7887, -62.2652)
  line L578 (56.7887, -62.2652) -> (56.8637, -62.3108)
  line L579 (56.8637, -62.3108) -> (56.939, -62.3545)
  line L580 (56.939, -62.3545) -> (57.0147, -62.3962)
  line L581 (57.0147, -62.3962) -> (57.0908, -62.4357)
  line L582 (57.0908, -62.4357) -> (57.1673, -62.4731)
  line L583 (57.1673, -62.4731) -> (57.2442, -62.5082)
  line L584 (57.2442, -62.5082) -> (57.3214, -62.5408)
  line L585 (57.3214, -62.5408) -> (57.3991, -62.5706)
  line L586 (57.3991, -62.5706) -> (57.4772, -62.5973)
  line L587 (57.4772, -62.5973) -> (57.5559, -62.6202)
  line L588 (57.5559, -62.6202) -> (57.6353, -62.6373)
  line L589 (57.6353, -62.6373) -> (57.9711, -62.6808)
  line L590 (57.9711, -62.6808) -> (57.9471, -62.8827)
  line L591 (57.9471, -62.8827) -> (57.9273, -63.085)
  line L592 (57.9273, -63.085) -> (57.9117, -63.2877)
  line L593 (57.9117, -63.2877) -> (57.9003, -63.4907)
  line L594 (57.9003, -63.4907) -> (57.562, -63.4752)
  line L595 (57.562, -63.4752) -> (57.4808, -63.4783)
  line L596 (57.4808, -63.4783) -> (57.3994, -63.4872)
  line L597 (57.3994, -63.4872) -> (57.3178, -63.4999)
  line L598 (57.3178, -63.4999) -> (57.2361, -63.5157)
  line L599 (57.2361, -63.5157) -> (57.1544, -63.5344)
  line L600 (57.1544, -63.5344) -> (57.0726, -63.5556)
  line L601 (57.0726, -63.5556) -> (56.9908, -63.5791)
  line L602 (56.9908, -63.5791) -> (56.909, -63.6049)
  line L603 (56.909, -63.6049) -> (56.8272, -63.6328)
  line L604 (56.8272, -63.6328) -> (56.7454, -63.6627)
  line L605 (56.7454, -63.6627) -> (56.6637, -63.6946)
  line L606 (56.6637, -63.6946) -> (56.582, -63.7284)
  line L607 (56.582, -63.7284) -> (56.5802, -63.8695)
  line L608 (56.5802, -63.8695) -> (56.5802, -64.0105)
  line L609 (56.5802, -64.0105) -> (56.582, -64.1516)
  line L610 (56.582, -64.1516) -> (56.6637, -64.1854)
  line L611 (56.6637, -64.1854) -> (56.7454, -64.2173)
  line L612 (56.7454, -64.2173) -> (56.8272, -64.2472)
  line L613 (56.8272, -64.2472) -> (56.909, -64.2751)
  line L614 (56.909, -64.2751) -> (56.9908, -64.3009)
  line L615 (56.9908, -64.3009) -> (57.0726, -64.3244)
  line L616 (57.0726, -64.3244) -> (57.1544, -64.3456)
  line L617 (57.1544, -64.3456) -> (57.2361, -64.3643)
  line L618 (57.2361, -64.3643) -> (57.3178, -64.3801)
  line L619 (57.3178, -64.3801) -> (57.3994, -64.3928)
  line L620 (57.3994, -64.3928) -> (57.4808, -64.4017)
  line L621 (57.4808, -64.4017) -> (57.562, -64.4048)
  line L622 (57.562, -64.4048) -> (57.9003, -64.3893)
  line L623 (57.9003, -64.3893) -> (57.9117, -64.5923)
  line L624 (57.9117, -64.5923) -> (57.9273, -64.795)
  line L625 (57.9273, -64.795) -> (57.9471, -64.9973)
  line L626 (57.9471, -64.9973) -> (57.9711, -65.1992)
  line L627 (57.9711, -65.1992) -> (57.6353, -65.2427)
  line L628 (57.6353, -65.2427) -> (57.5559, -65.2598)
  line L629 (57.5559, -65.2598) -> (57.4772, -65.2827)
  line L630 (57.4772, -65.2827) -> (57.3991, -65.3094)
  line L631 (57.3991, -65.3094) -> (57.3214, -65.3392)
  line L632 (57.3214, -65.3392) -> (57.2442, -65.3718)
  line L633 (57.2442, -65.3718) -> (57.1673, -65.4069)
  line L634 (57.1673, -65.4069) -> (57.0908, -65.4443)
  line L635 (57.0908, -65.4443) -> (57.0147, -65.4838)
  line L636 (57.0147, -65.4838) -> (56.939, -65.5255)
  line L637 (56.939, -65.5255) -> (56.8637, -65.5692)
  line L638 (56.8637, -65.5692) -> (56.7887, -65.6148)
  line L639 (56.7887, -65.6148) -> (56.7142, -65.6622)
  line L640 (56.7142, -65.6622) -> (56.7369, -65.8015)
  line L641 (56.7369, -65.8015) -> (56.7614, -65.9404)
  line L642 (56.7614, -65.9404) -> (56.7877, -66.079)
  line L643 (56.7877, -66.079) -> (56.874, -66.0981)
  line L644 (56.874, -66.0981) -> (56.96, -66.1153)
  line L645 (56.96, -66.1153) -> (57.0457, -66.1306)
  line L646 (57.0457, -66.1306) -> (57.1311, -66.1438)
  line L647 (57.1311, -66.1438) -> (57.2162, -66.155)
  line L648 (57.2162, -66.155) -> (57.3008, -66.164)
  line L649 (57.3008, -66.164) -> (57.385, -66.1707)
  line L650 (57.385, -66.1707) -> (57.4688, -66.1748)
  line L651 (57.4688, -66.1748) -> (57.552, -66.1763)
  line L652 (57.552, -66.1763) -> (57.6345, -66.1746)
  line L653 (57.6345, -66.1746) -> (57.7162, -66.1692)
  line L654 (57.7162, -66.1692) -> (57.7967, -66.1582)
  line L655 (57.7967, -66.1582) -> (58.1272, -66.0842)
  line L656 (58.1272, -66.0842) -> (58.1737, -66.2821)
  line L657 (58.1737, -66.2821) -> (58.2243, -66.479)
  line L658 (58.2243, -66.479) -> (58.2789, -66.6748)
  line L659 (58.2789, -66.6748) -> (58.3376, -66.8695)
  line L660 (58.3376, -66.8695) -> (58.0144, -66.9706)
  line L661 (58.0144, -66.9706) -> (57.9392, -67.0013)
  line L662 (57.9392, -67.0013) -> (57.8657, -67.0375)
  line L663 (57.8657, -67.0375) -> (57.7934, -67.0773)
  line L664 (57.7934, -67.0773) -> (57.7221, -67.1202)
  line L665 (57.7221, -67.1202) -> (57.6517, -67.1657)
  line L666 (57.6517, -67.1657) -> (57.582, -67.2136)
  line L667 (57.582, -67.2136) -> (57.5132, -67.2637)
  line L668 (57.5132, -67.2637) -> (57.4451, -67.3159)
  line L669 (57.4451, -67.3159) -> (57.3778, -67.3701)
  line L670 (57.3778, -67.3701) -> (57.3112, -67.4261)
  line L671 (57.3112, -67.4261) -> (57.2453, -67.484)
  line L672 (57.2453, -67.484) -> (57.1801, -67.5437)
  line L673 (57.1801, -67.5437) -> (57.2267, -67.6769)
  line L674 (57.2267, -67.6769) -> (57.275, -67.8095)
  line L675 (57.275, -67.8095) -> (57.3249, -67.9414)
  line L676 (57.3249, -67.9414) -> (57.4132, -67.9453)
  line L677 (57.4132, -67.9453) -> (57.5009, -67.9473)
  line L678 (57.5009, -67.9473) -> (57.5879, -67.9474)
  line L679 (57.5879, -67.9474) -> (57.6744, -67.9456)
  line L680 (57.6744, -67.9456) -> (57.7601, -67.9419)
  line L681 (57.7601, -67.9419) -> (57.845, -67.936)
  line L682 (57.845, -67.936) -> (57.9291, -67.9279)
  line L683 (57.9291, -67.9279) -> (58.0123, -67.9175)
  line L684 (58.0123, -67.9175) -> (58.0945, -67.9045)
  line L685 (58.0945, -67.9045) -> (58.1755, -67.8885)
  line L686 (58.1755, -67.8885) -> (58.255, -67.869)
  line L687 (58.255, -67.869) -> (58.3324, -67.8442)
  line L688 (58.3324, -67.8442) -> (58.645, -67.7139)
  line L689 (58.645, -67.7139) -> (58.7251, -67.9008)
  line L690 (58.7251, -67.9008) -> (58.8091, -68.0859)
  line L691 (58.8091, -68.0859) -> (58.8969, -68.2692)
  line L692 (58.8969, -68.2692) -> (58.9885, -68.4507)
  line L693 (58.9885, -68.4507) -> (58.6878, -68.6064)
  line L694 (58.6878, -68.6064) -> (58.6191, -68.6497)
  line L695 (58.6191, -68.6497) -> (58.553, -68.6981)
  line L696 (58.553, -68.6981) -> (58.4887, -68.7499)
  line L697 (58.4887, -68.7499) -> (58.4259, -68.8045)
  line L698 (58.4259, -68.8045) -> (58.3644, -68.8615)
  line L699 (58.3644, -68.8615) -> (58.3042, -68.9208)
  line L700 (58.3042, -68.9208) -> (58.2451, -68.9821)
  line L701 (58.2451, -68.9821) -> (58.1872, -69.0453)
  line L702 (58.1872, -69.0453) -> (58.1303, -69.1104)
  line L703 (58.1303, -69.1104) -> (58.0744, -69.1772)
  line L704 (58.0744, -69.1772) -> (58.0196, -69.2456)
  line L705 (58.0196, -69.2456) -> (57.9657, -69.3157)
  line L706 (57.9657, -69.3157) -> (58.0347, -69.4388)
  line L707 (58.0347, -69.4388) -> (58.1053, -69.561)
  line L708 (58.1053, -69.561) -> (58.1774, -69.6823)
  line L709 (58.1774, -69.6823) -> (58.265, -69.6707)
  line L710 (58.265, -69.6707) -> (58.3517, -69.6574)
  line L711 (58.3517, -69.6574) -> (58.4375, -69.6425)
  line L712 (58.4375, -69.6425) -> (58.5222, -69.6257)
  line L713 (58.5222, -69.6257) -> (58.606, -69.6071)
  line L714 (58.606, -69.6071) -> (58.6886, -69.5866)
  line L715 (58.6886, -69.5866) -> (58.77, -69.5641)
  line L716 (58.77, -69.5641) -> (58.8502, -69.5393)
  line L717 (58.8502, -69.5393) -> (58.9288, -69.5123)
  line L718 (58.9288, -69.5123) -> (59.0058, -69.4825)
  line L719 (59.0058, -69.4825) -> (59.0808, -69.4495)
  line L720 (59.0808, -69.4495) -> (59.1526, -69.4116)
  line L721 (59.1526, -69.4116) -> (59.4379, -69.229)
  line L722 (59.4379, -69.229) -> (59.5492, -69.3991)
  line L723 (59.5492, -69.3991) -> (59.6641, -69.5668)
  line L724 (59.6641, -69.5668) -> (59.7824, -69.7321)
  line L725 (59.7824, -69.7321) -> (59.9042, -69.8949)
  line L726 (59.9042, -69.8949) -> (59.635, -70.1005)
  line L727 (59.635, -70.1005) -> (59.5749, -70.1551)
  line L728 (59.5749, -70.1551) -> (59.5182, -70.2142)
  line L729 (59.5182, -70.2142) -> (59.4639, -70.2764)
  line L730 (59.4639, -70.2764) -> (59.4115, -70.341)
  line L731 (59.4115, -70.341) -> (59.3609, -70.4079)
  line L732 (59.3609, -70.4079) -> (59.3119, -70.4767)
  line L733 (59.3119, -70.4767) -> (59.2643, -70.5473)
  line L734 (59.2643, -70.5473) -> (59.2182, -70.6196)
  line L735 (59.2182, -70.6196) -> (59.1735, -70.6936)
  line L736 (59.1735, -70.6936) -> (59.1301, -70.7691)
  line L737 (59.1301, -70.7691) -> (59.0879, -70.846)
  line L738 (59.0879, -70.846) -> (59.0471, -70.9244)
  line L739 (59.0471, -70.9244) -> (59.1364, -71.0336)
  line L740 (59.1364, -71.0336) -> (59.2271, -71.1417)
  line L741 (59.2271, -71.1417) -> (59.3192, -71.2486)
  line L742 (59.3192, -71.2486) -> (59.4034, -71.222)
  line L743 (59.4034, -71.222) -> (59.4865, -71.1939)
  line L744 (59.4865, -71.1939) -> (59.5684, -71.1642)
  line L745 (59.5684, -71.1642) -> (59.649, -71.133)
  line L746 (59.649, -71.133) -> (59.7282, -71.1002)
  line L747 (59.7282, -71.1002) -> (59.806, -71.0656)
  line L748 (59.806, -71.0656) -> (59.8823, -71.0293)
  line L749 (59.8823, -71.0293) -> (59.9569, -70.991)
  line L750 (59.9569, -70.991) -> (60.0297, -70.9507)
  line L751 (60.0297, -70.9507) -> (60.1003, -70.908)
  line L752 (60.1003, -70.908) -> (60.1684, -70.8625)
  line L753 (60.1684, -70.8625) -> (60.2326, -70.8127)
  line L754 (60.2326, -70.8127) -> (60.4818, -70.5833)
  line L755 (60.4818, -70.5833) -> (60.621, -70.7315)
  line L756 (60.621, -70.7315) -> (60.7633, -70.8767)
  line L757 (60.7633, -70.8767) -> (60.9085, -71.019)
  line L758 (60.9085, -71.019) -> (61.0567, -71.1582)
  line L759 (61.0567, -71.1582) -> (60.8273, -71.4074)
  line L760 (60.8273, -71.4074) -> (60.7775, -71.4716)
  line L761 (60.7775, -71.4716) -> (60.732, -71.5397)
  line L762 (60.732, -71.5397) -> (60.6893, -71.6103)
  line L763 (60.6893, -71.6103) -> (60.649, -71.6831)
  line L764 (60.649, -71.6831) -> (60.6107, -71.7577)
  line L765 (60.6107, -71.7577) -> (60.5744, -71.834)
  line L766 (60.5744, -71.834) -> (60.5398, -71.9118)
  line L767 (60.5398, -71.9118) -> (60.507, -71.991)
  line L768 (60.507, -71.991) -> (60.4758, -72.0716)
  line L769 (60.4758, -72.0716) -> (60.4461, -72.1535)
  line L770 (60.4461, -72.1535) -> (60.418, -72.2366)
  line L771 (60.418, -72.2366) -> (60.3914, -72.3208)
  line L772 (60.3914, -72.3208) -> (60.4983, -72.4129)
  line L773 (60.4983, -72.4129) -> (60.6064, -72.5036)
  line L774 (60.6064, -72.5036) -> (60.7156, -72.5929)
  line L775 (60.7156, -72.5929) -> (60.794, -72.5521)
  line L776 (60.794, -72.5521) -> (60.8709, -72.5099)
  line L777 (60.8709, -72.5099) -> (60.9464, -72.4665)
  line L778 (60.9464, -72.4665) -> (61.0204, -72.4218)
  line L779 (61.0204, -72.4218) -> (61.0927, -72.3757)
  line L780 (61.0927, -72.3757) -> (61.1633, -72.3281)
  line L781 (61.1633, -72.3281) -> (61.2321, -72.2791)
  line L782 (61.2321, -72.2791) -> (61.299, -72.2285)
  line L783 (61.299, -72.2285) -> (61.3636, -72.1761)
  line L784 (61.3636, -72.1761) -> (61.4258, -72.1218)
  line L785 (61.4258, -72.1218) -> (61.4849, -72.0651)
  line L786 (61.4849, -72.0651) -> (61.5395, -72.005)
  line L787 (61.5395, -72.005) -> (61.7451, -71.7358)
  line L788 (61.7451, -71.7358) -> (61.9079, -71.8576)
  line L789 (61.9079, -71.8576) -> (62.0732, -71.9759)
  line L790 (62.0732, -71.9759) -> (62.2409, -72.0908)
  line L791 (62.2409, -72.0908) -> (62.411, -72.2021)
  line L792 (62.411, -72.2021) -> (62.2284, -72.4874)
  line L793 (62.2284, -72.4874) -> (62.1905, -72.5592)
  line L794 (62.1905, -72.5592) -> (62.1575, -72.6342)
  line L795 (62.1575, -72.6342) -> (62.1277, -72.7112)
  line L796 (62.1277, -72.7112) -> (62.1007, -72.7898)
  line L797 (62.1007, -72.7898) -> (62.0759, -72.87)
  line L798 (62.0759, -72.87) -> (62.0534, -72.9514)
  line L799 (62.0534, -72.9514) -> (62.0329, -73.034)
  line L800 (62.0329, -73.034) -> (62.0143, -73.1178)
  line L801 (62.0143, -73.1178) -> (61.9975, -73.2025)
  line L802 (61.9975, -73.2025) -> (61.9826, -73.2883)
  line L803 (61.9826, -73.2883) -> (61.9693, -73.375)
  line L804 (61.9693, -73.375) -> (61.9577, -73.4626)
  line L805 (61.9577, -73.4626) -> (62.079, -73.5347)
  line L806 (62.079, -73.5347) -> (62.2012, -73.6053)
  line L807 (62.2012, -73.6053) -> (62.3243, -73.6743)
  line L808 (62.3243, -73.6743) -> (62.3944, -73.6204)
  line L809 (62.3944, -73.6204) -> (62.4628, -73.5656)
  line L810 (62.4628, -73.5656) -> (62.5296, -73.5097)
  line L811 (62.5296, -73.5097) -> (62.5947, -73.4528)
  line L812 (62.5947, -73.4528) -> (62.6579, -73.3949)
  line L813 (62.6579, -73.3949) -> (62.7192, -73.3358)
  line L814 (62.7192, -73.3358) -> (62.7785, -73.2756)
  line L815 (62.7785, -73.2756) -> (62.8355, -73.2141)
  line L816 (62.8355, -73.2141) -> (62.8901, -73.1513)
  line L817 (62.8901, -73.1513) -> (62.9419, -73.087)
  line L818 (62.9419, -73.087) -> (62.9903, -73.0209)
  line L819 (62.9903, -73.0209) -> (63.0336, -72.9522)